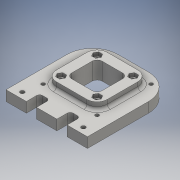
# Autodesk Inventor part: mbot_rear_UTM-30LX_mount
Saved by Autodesk Inventor 2016 (Build 200138000, 138)
## iProperties
Created: 2016-10-09
Part Number: mbot_rear_UTM-30LX_mount
Material: Generic
Document SubType Name: Modeling
Designer: oscar
Density: 1 g/cm^3
Appearance: Default
Author: oscar
Autodesk Inventor part; units mm, degrees
ref_plane "YZ Plane" through (0, 0, 0) normal (1, 0, 0) x (0, 1, 0)
ref_plane "XZ Plane" through (0, 0, 0) normal (0, 1, 0) x (-1, 0, 0)
ref_plane "XY Plane" through (0, 0, 0) normal (0, 0, 1) x (1, 0, 0)
sketch "Sketch1" plane through (0, 0, 0) normal (0, 0, 1) x (1, 0, 0)
  line L0 (10.3456, 14.8047) -> (30.3456, 14.8047)
  line L1 (40.3456, 14.8047) -> (60.3456, 14.8047)
  line L2 (70.3456, 14.8047) -> (90.3456, 14.8047)
  circle A0 centre (20.3456, 20.8047) radius 2
  circle A1 centre (80.3456, 20.8047) radius 2
  circle A2 centre (23.8456, 90.8047) radius 1.75
  circle A3 centre (76.8456, 90.8047) radius 1.75
  circle A4 centre (76.8456, 37.8047) radius 1.75
  circle A5 centre (23.8456, 37.8047) radius 1.75
  arc A6 (75.3456, 79.3047) -> (65.3456, 89.3047) centre (65.3456, 79.3047) ccw
  arc A7 (35.3456, 89.3047) -> (25.3456, 79.3047) centre (35.3456, 79.3047) ccw
  arc A8 (65.3456, 39.3047) -> (75.3456, 49.3047) centre (65.3456, 49.3047) ccw
  arc A9 (25.3456, 49.3047) -> (35.3456, 39.3047) centre (35.3456, 49.3047) ccw
  arc A10 (40.3456, 79.3047) -> (35.3456, 74.3047) centre (40.3456, 74.3047) ccw
  arc A11 (65.3456, 74.3047) -> (60.3456, 79.3047) centre (60.3456, 74.3047) ccw
  arc A12 (35.3456, 54.3047) -> (40.3456, 49.3047) centre (40.3456, 54.3047) ccw
  arc A13 (60.3456, 49.3047) -> (65.3456, 54.3047) centre (60.3456, 54.3047) ccw
  arc A14 (33.3456, 27.8047) -> (30.3456, 24.8047) centre (33.3456, 24.8047) ccw
  arc A15 (40.3456, 24.8047) -> (37.3456, 27.8047) centre (37.3456, 24.8047) ccw
  arc A16 (63.3456, 27.8047) -> (60.3456, 24.8047) centre (63.3456, 24.8047) ccw
  arc A17 (70.3456, 24.8047) -> (67.3456, 27.8047) centre (67.3456, 24.8047) ccw
  line L3 (34.668, 78.5182) -> (36.668, 81.9823)
  line L4 (34.668, 85.4464) -> (30.668, 85.4464)
  line L5 (28.668, 81.9823) -> (30.668, 78.5182)
  line L6 (70.0233, 78.5182) -> (72.0233, 81.9823)
  line L7 (70.0233, 85.4464) -> (66.0233, 85.4464)
  line L8 (64.0233, 81.9823) -> (66.0233, 78.5182)
  line L9 (70.0233, 43.1629) -> (72.0233, 46.627)
  line L10 (70.0233, 50.0911) -> (66.0233, 50.0911)
  line L11 (64.0233, 46.627) -> (66.0233, 43.1629)
  line L12 (34.668, 43.1629) -> (36.668, 46.627)
  line L13 (34.668, 50.0911) -> (30.668, 50.0911)
  line L14 (28.668, 46.627) -> (30.668, 43.1629)
  arc A18 (35.3456, 99.8047) -> (10.3456, 74.8047) centre (35.3456, 74.8047) ccw
  arc A19 (90.3456, 74.8047) -> (65.3456, 99.8047) centre (65.3456, 74.8047) ccw
  line L15 (10.3456, 74.8047) -> (10.3456, 14.8047)
  line L16 (30.3456, 14.8047) -> (30.3456, 24.8047)
  line L17 (33.3456, 27.8047) -> (37.3456, 27.8047)
  line L18 (40.3456, 14.8047) -> (40.3456, 24.8047)
  line L19 (60.3456, 14.8047) -> (60.3456, 24.8047)
  line L20 (63.3456, 27.8047) -> (67.3456, 27.8047)
  line L21 (70.3456, 24.8047) -> (70.3456, 14.8047)
  line L22 (90.3456, 14.8047) -> (90.3456, 74.8047)
  line L23 (35.3456, 99.8047) -> (65.3456, 99.8047)
  line L24 (35.3456, 89.3047) -> (65.3456, 89.3047)
  line L25 (75.3456, 79.3047) -> (75.3456, 49.3047)
  line L26 (65.3456, 39.3047) -> (35.3456, 39.3047)
  line L27 (25.3456, 49.3047) -> (25.3456, 79.3047)
  line L28 (30.668, 85.4464) -> (28.668, 81.9823)
  line L29 (34.668, 85.4464) -> (36.668, 81.9823)
  line L30 (34.668, 78.5182) -> (30.668, 78.5182)
  line L31 (64.0233, 81.9823) -> (66.0233, 85.4464)
  line L32 (70.0233, 85.4464) -> (72.0233, 81.9823)
  line L33 (70.0233, 78.5182) -> (66.0233, 78.5182)
  line L34 (30.668, 50.0911) -> (28.668, 46.627)
  line L35 (30.668, 43.1629) -> (34.668, 43.1629)
  line L36 (36.668, 46.627) -> (34.668, 50.0911)
  line L37 (64.0233, 46.627) -> (66.0233, 50.0911)
  line L38 (70.0233, 50.0911) -> (72.0233, 46.627)
  line L39 (70.0233, 43.1629) -> (66.0233, 43.1629)
  circle A20 centre (32.668, 81.9823) radius 2
  circle A21 centre (68.0233, 81.9823) radius 2
  circle A22 centre (68.0233, 46.627) radius 2
  circle A23 centre (32.668, 46.627) radius 2
  line L40 (35.3456, 74.3047) -> (35.3456, 54.3047)
  line L41 (40.3456, 49.3047) -> (60.3456, 49.3047)
  line L42 (65.3456, 54.3047) -> (65.3456, 74.3047)
  line L43 (60.3456, 79.3047) -> (40.3456, 79.3047)
  point P0 (0, 0)
  dimension "d0" = 4
  dimension "d1" = 4
  dimension "d2" = 4
  dimension "d3" = 4
  constraints: 88 end point, 28 point on circle, 24 centre point, 12 perpendicular, 8 parallel, 2 collinear, 2 tangent, 2 vertical, 1 horizontal
  measures "d0" diameter of A20
  measures "d1" diameter of A21
  measures "d2" diameter of A22
  measures "d3" diameter of A23
extrude "Extrusion1" add sketch "Sketch1" along normal blind 10 contours L15 A18 L23 A19 L22 L2 L21 A17 L20 A16 L19 L1 L18 A15 L17 A14 L16 L0
extrude "Extrusion3" add sketch "Sketch1" along normal blind 17 contours L25 A8 L26 A9 L27 A7 L24 A6
extrude "Extrusion4" add sketch "Sketch1" along normal blind 13.5 contours L30 L5 L28 L4 L29 L3 | L33 L8 L31 L7 L32 L6 | L39 L11 L37 L10 L38 L9 | L35 L14 L34 L13 L36 L12
fillet "Fillet1" radius 3 8 edges at (72.4167, 42.2336, 10) (50.3456, 39.3047, 10) (28.2746, 42.2336, 10) (25.3456, 64.3047, 10) (28.2746, 86.3757, 10) (50.3456, 89.3047, 10) (72.4167, 86.3757, 10) (75.3456, 64.3047, 10)
chamfer "Chamfer1" distance 2 angle 45 4 edges at (75.0956, 90.8047, 0) (22.0956, 90.8047, 0) (75.0956, 37.8047, 0) (22.0956, 37.8047, 0)
chamfer "Chamfer2" distance 2.5 angle 45 2 edges at (78.3456, 20.8047, 0) (18.3456, 20.8047, 0)
body "Solid1"
